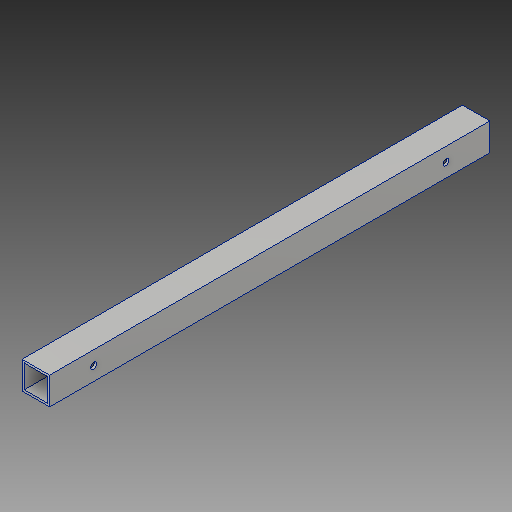
# Autodesk Inventor part: Top Support
Saved by Autodesk Inventor 2019.4 (Build 234330000, 330)
## iProperties
Created: 2020-01-10
Part Number: Top Support
Material: Aluminum 6061
Document SubType Name: Modeling
Designer: Mark
Mass: 198.207 g
Surface Area: 739.162 cm^2
Volume: 73.4099 cm^3
Density: 2.7 g/cm^3
Appearance: Aluminum - Flat
Author: Mark
Autodesk Inventor part; units mm, degrees
ref_plane "YZ Plane" through (0, 0, 0) normal (1, 0, 0) x (0, 1, 0)
ref_plane "XZ Plane" through (0, 0, 0) normal (0, 1, 0) x (-1, 0, 0)
ref_plane "XY Plane" through (0, 0, 0) normal (0, 0, 1) x (1, 0, 0)
sketch "Sketch1" plane through (0, 0, 0) normal (0, 0, 1) x (1, 0, 0)
  line L0 (-12.5, -12.5) -> (12.5, -12.5)
  line L1 (12.5, -12.5) -> (12.5, 12.5)
  line L2 (12.5, 12.5) -> (-12.5, 12.5)
  line L3 (-12.5, 12.5) -> (-12.5, -12.5)
  line L4 (-12.5, -12.5) -> (12.5, 12.5) construction
  line L5 (12.5, -12.5) -> (-12.5, 12.5) construction
  line L6 (-10.5, -10.5) -> (10.5, -10.5)
  line L7 (10.5, -10.5) -> (10.5, 10.5)
  line L8 (10.5, 10.5) -> (-10.5, 10.5)
  line L9 (-10.5, 10.5) -> (-10.5, -10.5)
  line L10 (-10.5, -10.5) -> (10.5, 10.5) construction
  line L11 (10.5, -10.5) -> (-10.5, 10.5) construction
  point P0 (0, 0)
  dimension "d0" = 25
  dimension "d1" = 25
  dimension "d2" = 21
  dimension "d3" = 21
  constraints: 24 end point, 4 midpoint, 4 parallel, 2 horizontal, 2 perpendicular
  measures "d0" distance of L2.end L1.end
  measures "d1" distance of L1.end L0.end
  measures "d2" distance of L8.end L7.end
  measures "d3" distance of L7.end L6.end
extrude "Extrusion1" add sketch "Sketch1" along normal blind 400
sketch "Sketch2" plane through (12.5, -12.5, 0) normal (1, 0, 0) x (0, 0, -1)
  circle A0 centre (-360, 12.5) radius 2.75
  circle A1 centre (-40, 12.5) radius 2.75
  line L0 (0, 0) -> (0, 25) projected
  line L1 (0, 25) -> (-400, 25) projected
  line L2 (-400, 0) -> (-400, 25) projected
  point P0 (0, 12.5)
  dimension "d6" = 5.5
  dimension "d7" = 5.5
  dimension "d8" = 40
  dimension "d9" = 12.5
  dimension "d10" = 40
  dimension "d11" = 12.5
  constraints: 2 centre point
  measures "d6" diameter of A0
  measures "d7" diameter of A1
  measures "d8" distance from line of L0 A1.centre
  measures "d9" distance from line of L1 A1.centre
  measures "d10" distance from line of L2 A0.centre
  measures "d11" distance from line of L1 A0.centre
extrude "Extrusion2" cut sketch "Sketch2" against normal blind 25
body "Solid1"
